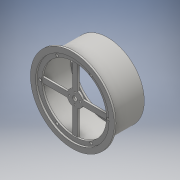
# Autodesk Inventor part: Motor mount (plain)
Saved by Autodesk Inventor 2016 (Build 200138000, 138)
## iProperties
Created: 2016-03-10
Part Number: Motor mount (plain)
Material: Generic
Document SubType Name: Modeling
Designer: s_sud
Density: 1 g/cm^3
Appearance: Default
Author: s_sud
Autodesk Inventor part; units mm, degrees
ref_plane "YZ Plane" through (0, 0, 0) normal (1, 0, 0) x (0, 1, 0)
ref_plane "XZ Plane" through (0, 0, 0) normal (0, 1, 0) x (-1, 0, 0)
ref_plane "XY Plane" through (0, 0, 0) normal (0, 0, 1) x (1, 0, 0)
sketch "Sketch1" plane through (0, 0, 0) normal (0, 1, 0) x (-1, 0, 0)
  circle A0 centre (0, 0) radius 40
  circle A1 centre (0, 0) radius 41.5
  dimension "d0" = 80
  dimension "d1" = 83
  constraints: 2 centre point, 2 coincident
  measures "d0" diameter of A0
  measures "d1" diameter of A1
extrude "Extrusion1" add sketch "Sketch1" along normal blind 35
sketch "Sketch7" plane through (0, 0, 0) normal (0, -1, 0) x (1, 0, 0)
  line L0 (-3, -41) -> (3, -41)
  line L1 (3, 41) -> (-3, 41)
  line L2 (-3, -41) -> (3, 41) construction
  line L3 (3, -41) -> (-3, 41) construction
  line L4 (41, -3) -> (41, 3)
  line L5 (-41, 3) -> (-41, -3)
  line L6 (-41, -3) -> (41, 3) construction
  line L7 (41, -3) -> (-41, 3) construction
  line L8 (-3, 41) -> (-3, 8.4853)
  line L9 (-8.4853, 3) -> (-41, 3)
  line L10 (3, 8.4853) -> (3, 41)
  line L11 (41, 3) -> (8.4853, 3)
  line L12 (-3, -8.4853) -> (-3, -41)
  line L13 (-41, -3) -> (-8.4853, -3)
  line L14 (3, -41) -> (3, -8.4853)
  line L15 (8.4853, -3) -> (41, -3)
  arc A0 (3, -8.4853) -> (8.4853, -3) centre (0, 0) ccw
  arc A1 (-8.4853, -3) -> (-3, -8.4853) centre (0, 0) ccw
  arc A2 (8.4853, 3) -> (3, 8.4853) centre (0, 0) ccw
  arc A3 (-3, 8.4853) -> (-8.4853, 3) centre (0, 0) ccw
  circle A4 centre (0, 6) radius 1
  circle A5 centre (-6, 0) radius 1
  circle A6 centre (0, -6) radius 1
  circle A7 centre (6, 0) radius 1
  circle A8 centre (0, 0) radius 2.6207
  dimension "d35" = 6
  dimension "d36" = 82
  dimension "d37" = 6
  dimension "d38" = 82
  dimension "d41" = 2
  dimension "d44" = 360
  constraints: 32 end point, 10 parallel, 9 centre point, 8 point on circle, 4 midpoint, 4 perpendicular, 3 horizontal, 2 coincident, 9 other
  measures "d35" distance of L1.end L1.start
  measures "d36" distance of L0.end L1.start
  measures "d37" distance of L4.start L4.end
  measures "d38" distance of L5.end L4.start
  measures "d41" diameter of A4
extrude "Extrusion7" add sketch "Sketch7" along normal blind 2
sketch "Sketch8" plane through (0, 0, 0) normal (0, -1, 0) x (1, 0, 0)
  circle A0 centre (0, 0) radius 41.5606
  circle A1 centre (0, 0) radius 40
  circle A2 centre (0, 0) radius 41.5606
  circle A3 centre (0, 0) radius 40
  constraints: 4 centre point, 4 coincident, 2 concentric
extrude "Extrusion8" add sketch "Sketch8" along normal blind 3
sketch "Sketch9" plane through (0, -3, 0) normal (0, -1, 0) x (1, 0, 0)
  circle A0 centre (0, 0) radius 36.6376
  circle A1 centre (0, 0) radius 41.5606 projected
  constraints: 1 centre point, 1 coincident
extrude "Extrusion9" add sketch "Sketch9" against normal blind 2
sketch "Sketch10" plane through (0, 35, 0) normal (0, 1, 0) x (1, 0, 0)
  circle A0 centre (0, 0) radius 36.5
  circle A1 centre (0, 0) radius 41.5
  dimension "d52" = 73
  dimension "d53" = 83
  constraints: 2 centre point, 2 coincident
  measures "d52" diameter of A0
  measures "d53" diameter of A1
extrude "Extrusion10" add sketch "Sketch10" against normal blind 2
sketch "Sketch11" plane through (0, 35, 0) normal (0, 1, 0) x (1, 0, 0)
  circle A0 centre (-38.5, 0) radius 1.5
  circle A1 centre (-19.25, -33.342) radius 1.5
  circle A2 centre (19.25, -33.342) radius 1.5
  circle A3 centre (38.5, 0) radius 1.5
  circle A4 centre (19.25, 33.342) radius 1.5
  circle A5 centre (-19.25, 33.342) radius 1.5
  point P0 (0, 0)
  dimension "d56" = 3
  dimension "d57" = 38.5
  dimension "d60" = 360
  constraints: 6 centre point, 13 other
  measures "d56" diameter of A0
  measures "d57" distance of point (0, 0) A0.centre
extrude "Extrusion11" cut sketch "Sketch11" against normal blind 100
sketch "Sketch12" plane through (0, -3, 0) normal (0, -1, 0) x (1, 0, 0)
  circle A0 centre (0, 0) radius 47.5
  circle A1 centre (0, 0) radius 41.5606 projected
  dimension "d64" = 95
  constraints: 1 centre point, 1 coincident
  measures "d64" diameter of A0
extrude "Extrusion12" add sketch "Sketch12" along normal blind 2
body "Solid1"
